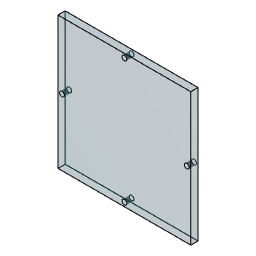
кубсат 2.0 v4 (Autodesk Fusion 360 archive; units mm, degrees)
design "стекло на кубсат 2.0"
Autodesk Fusion 360 part; units mm, degrees
sketch "Sketch1" plane through (0, 0, 0) normal (0, 1, 0) x (1, 0, 0)
  line L0 (-50, -50) -> (33, -50)
  line L1 (33, -50) -> (33, 33)
  line L2 (33, 33) -> (-50, 33)
  line L3 (-50, 33) -> (-50, -50)
  line L4 (-50, -50) -> (-47.5, -50)
  line L5 (-47.5, -50) -> (-47.5, -47.5)
  line L6 (-47.5, -47.5) -> (-50, -47.5)
  line L7 (-50, -47.5) -> (-50, -50)
  line L8 (33, 33) -> (30.5, 33)
  line L9 (30.5, 33) -> (30.5, 30.5)
  line L10 (30.5, 30.5) -> (33, 30.5)
  line L11 (33, 30.5) -> (33, 33)
  line L12 (-47.5, -47.5) -> (30.5, -47.5)
  line L13 (30.5, -47.5) -> (30.5, 30.5)
  line L14 (30.5, 30.5) -> (-47.5, 30.5)
  line L15 (-47.5, 30.5) -> (-47.5, -47.5)
  circle A0 centre (-8.5, -47.5) radius 1.5
  circle A1 centre (-47.5, -8.5) radius 1.5
  circle A2 centre (-8.5, 30.5) radius 1.5
  circle A3 centre (30.5, -8.5) radius 1.5
  dimension "d1" = 83
  dimension "d2" = 83
  dimension "d3" = 2.5
  dimension "d4" = 2.5
  dimension "d5" = 2.5
  dimension "d6" = 2.5
  dimension "d7" = 3
  dimension "d8" = 3
  dimension "d9" = 3
  dimension "d10" = 3
  constraint horizontal L0
  constraint vertical L1
  constraint horizontal L2
  constraint vertical L3
  constraint horizontal L4
  constraint vertical L5
  constraint horizontal L6
  constraint vertical L7
  constraint horizontal L8
  constraint vertical L9
  constraint horizontal L10
  constraint vertical L11
  constraint horizontal L12
  constraint vertical L13
  constraint horizontal L14
  constraint vertical L15
  constraint midpoint L12 A0.centre
  constraint midpoint L15 A1.centre
  constraint midpoint L14 A2.centre
  constraint midpoint L13 A3.centre
  measures "d1" distance of L0.start L0.end
  measures "d2" distance of L0.start L2.end
  measures "d3" distance of L0.start L4.end
  measures "d4" distance of L0.start L6.end
  measures "d5" distance of L1.end L8.end
  measures "d6" distance of L1.end L10.end
  measures "d7" diameter of A0
  measures "d8" diameter of A1
  measures "d9" diameter of A2
  measures "d10" diameter of A3
extrude "Extrude1" add sketch "Sketch1" along normal blind 4.5 contours L0 L3 L4 L5 L6 L7 | L0 L1 L5 L10 L12 L13 A0 A3 | L2 L3 L6 L9 L14 L15 A1 A2 | L12 L13 L14 L15 A0 A1 A2 A3 | L1 L2 L8 L9 L10 L11

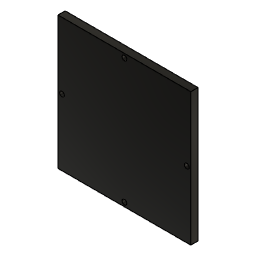
design "стена кубсата"
Autodesk Fusion 360 part; units mm, degrees
sketch "Sketch1" plane through (0, 0, 0) normal (0, 1, 0) x (1, 0, 0)
  line L0 (0, 0) -> (83, 0)
  line L1 (83, 0) -> (83, -83)
  line L2 (83, -83) -> (0, -83)
  line L3 (0, -83) -> (0, 0)
  line L4 (5, -78) -> (78, -78)
  line L5 (78, -78) -> (78, -5)
  line L6 (78, -5) -> (5, -5)
  line L7 (5, -5) -> (5, -78)
  line L8 (5, -78) -> (5, -80.5)
  line L9 (0, -80.5) -> (83, -80.5)
  circle A0 centre (41.5, -80.5) radius 1.5
  line L10 (0, -41.5) -> (26, -41.5)
  line L11 (0, -83) -> (13, -70)
  circle A1 centre (2.5, -41.5) radius 1.5
  line L12 (41.5, -80.5) -> (41.5, -76)
  circle A2 centre (80.5, -41.5) radius 1.5
  circle A3 centre (41.5, -2.5) radius 1.5
  dimension "d1" = 83
  dimension "d2" = 83
  dimension "d3" = 2.5
  dimension "d4" = 3
  constraint horizontal L0
  constraint vertical L1
  constraint horizontal L2
  constraint vertical L3
  constraint coincident L0.start L3.end
  constraint horizontal L4
  constraint vertical L5
  constraint horizontal L6
  constraint vertical L7
  constraint perpendicular L2 L8
  constraint coincident L3 L9.start
  constraint coincident L1 L9.end
  constraint perpendicular L1 L9
  constraint midpoint L9 A0.centre
  constraint midpoint L3 L10.start
  constraint perpendicular L3 L10
  constraint symmetric A0 L11 A1
  constraint coincident A0.centre L12.start
  constraint perpendicular L4 L12
  constraint symmetric A1 L12 A2
  constraint symmetric A0 L10 A3
  measures "d1" distance of L0.start L0.end
  measures "d2" distance of L0.start L2.end
  measures "d3" distance of L4.start L8.end
  measures "d4" diameter of A0
extrude "Extrude1" add sketch "Sketch1" along normal blind 4.5 contours L0 L1 L3 L4 L5 L6 L7 L9 A0 L10 A1 L12 | L3 L7 L9 L10 L11 A1 | L1 L2 L9 A0 L11 | L3 L9 L11 | L8 L9 L11 | L4 L8 L9 A0 L12 | L4 L5 L6 L7

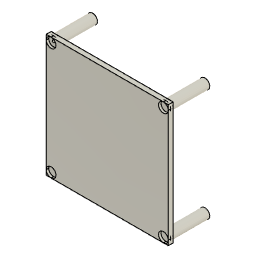
design "Untitled"
Autodesk Fusion 360 part; units mm, degrees
sketch "Sketch1" plane through (0, 0, 0) normal (0, 1, 0) x (1, 0, 0)
  line L0 (-60, -70) -> (-14, -70)
  line L1 (-14, -70) -> (-14, -24)
  line L2 (-14, -24) -> (-60, -24)
  line L3 (-60, -24) -> (-60, -70)
  circle A0 centre (-60, -70) radius 2
  circle A1 centre (-14, -70) radius 2
  circle A2 centre (-60, -24) radius 2
  circle A3 centre (-14, -24) radius 2
  dimension "d1" = 46
  dimension "d2" = 46
  dimension "d3" = 4
  dimension "d4" = 4
  dimension "d5" = 4
  dimension "d6" = 4
  constraint horizontal L0
  constraint vertical L1
  constraint horizontal L2
  constraint vertical L3
  constraint coincident L0.start L3.end
  constraint coincident L0.end L1.start
  constraint coincident L2.end L3.start
  constraint coincident L1.end L2.start
  measures "d1" distance of L0.start L0.end
  measures "d2" distance of L0.start L2.end
  measures "d3" diameter of A0
  measures "d4" diameter of A1
  measures "d5" diameter of A2
  measures "d6" diameter of A3
extrude "Extrude1" add sketch "Sketch1" against normal blind 15 contours L0 L3 A0 | L0 L3 A0 | L0 L1 A1 | L0 L1 A1 | L2 L3 A2 | L2 L3 A2 | L1 L2 A3 | L1 L2 A3 makes body 1 at (-12.1206, -10, 69.316) makes body 2 at (-58.0099, -5, 23.8009) makes body 3 at (-58.0618, -5, 69.5065) makes body 4 at (-12.0099, -10, 24.1991)
sketch "Sketch2" plane through (0, -15, 0) normal (0, -1, 0) x (1, 0, 0)
  circle A0 centre (-60, 70) radius 2
  line L0 (-62, 72) -> (-12, 72)
  line L1 (-12, 72) -> (-12, 22)
  line L2 (-12, 22) -> (-62, 22)
  line L3 (-62, 22) -> (-62, 72)
  constraint horizontal L0
  constraint vertical L1
  constraint horizontal L2
  constraint vertical L3
extrude "Extrude2" add sketch "Sketch2" along normal blind 2 bodies 1 2 3 4
sketch "Sketch3" plane through (0, -17, 0) normal (0, -1, 0) x (1, 0, 0)
  line L0 (-62, 22) -> (-12, 22)
  line L1 (-12, 22) -> (-12, 72)
  line L2 (-12, 72) -> (-62, 72)
  line L3 (-62, 72) -> (-62, 22)
  line L4 (-62, 72) -> (-12, 22)
  line L5 (-62, 72) -> (-59.1716, 69.1716)
  circle A0 centre (-60.5, 70.5) radius 1.5
  circle A1 through (-59.5, 70, -17) (-60.25, 70.433, -17) (-60.25, 69.567, -17)
  dimension "d11" = 4
  dimension "d12" = 1
  constraint coincident L2.end L3.start
  constraint coincident L0.end L1.start
  constraint parallel L4 L5
  constraint coincident L5 A0.centre
  constraint tangent L2 A0
  measures "d11" distance of L2.end L5.end
extrude "Extrude3" cut sketch "Sketch3" along normal blind 59 contours A1 in plane through (0, 0, 0) normal (0, -1, 0) bodies 1
sketch "Sketch4" plane through (0, -17, 0) normal (0, -1, 0) x (1, 0, 0)
  circle A0 centre (-60, 70) radius 0.5
  line L0 (-62, 22) -> (-12, 22)
  line L1 (-12, 22) -> (-12, 72)
  line L2 (-12, 72) -> (-62, 72)
  line L3 (-62, 72) -> (-62, 22)
  circle A1 centre (-60, 70) radius 2
  dimension "d15" = 4
  constraint concentric A0 A1
  measures "d15" diameter of A1
extrude "Extrude4" cut sketch "Sketch4" against normal blind 1 contours A1 bodies 1
sketch "Sketch5" plane through (0, -17, 0) normal (0, -1, 0) x (1, 0, 0)
  arc A0 (-62, 70) -> (-60, 72) centre (-60, 70) ccw
  line L0 (-62, 70) -> (-62, 22)
  line L1 (-62, 22) -> (-12, 22)
  line L2 (-12, 22) -> (-12, 72)
  line L3 (-12, 72) -> (-60, 72)
  circle A1 centre (-60, 70) radius 2
  line L4 (-62, 72) -> (-37, 72)
  line L5 (-37, 72) -> (-37, 61.6718)
  circle A2 centre (-14, 70) radius 2
  line L6 (-62, 72) -> (-62, 47)
  line L7 (-62, 47) -> (-51.7129, 47)
  circle A3 centre (-60, 24) radius 2
  circle A4 centre (-14, 24) radius 2
  dimension "d18" = 25
  dimension "d19" = 25
  constraint concentric A0 A1
  constraint perpendicular L3 L5
  constraint symmetric A1 L5 A2
  constraint perpendicular L0 L7
  constraint symmetric A1 L7 A3
  constraint symmetric A2 L7 A4
  measures "d18" distance of L4.start L4.end
  measures "d19" distance of L4.start L6.end
extrude "Extrude5" cut sketch "Sketch5" against normal blind 1 contours A3 | A2 | A4 bodies 1

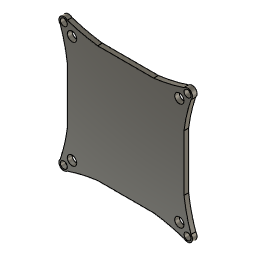
design "основа картриджа под кубсат 2.0"
Autodesk Fusion 360 part; units mm, degrees
sketch "Sketch1" plane through (0, 0, 0) normal (0, 1, 0) x (1, 0, 0)
  line L0 (0, 0) -> (50, 0)
  line L1 (50, 0) -> (50, -50)
  line L2 (50, -50) -> (0, -50)
  line L3 (0, -50) -> (0, 0)
  line L4 (0, -50) -> (-3, -50)
  line L5 (-3, -50) -> (-3, -53)
  line L6 (-3, -53) -> (0, -53)
  line L7 (0, -53) -> (0, -50)
  line L8 (50, 0) -> (53, 0)
  line L9 (53, 0) -> (53, 3)
  line L10 (53, 3) -> (50, 3)
  line L11 (50, 3) -> (50, 0)
  line L12 (0, 0) -> (-3, 0)
  line L13 (-3, 0) -> (-3, 3)
  line L14 (-3, 3) -> (0, 3)
  line L15 (0, 3) -> (0, 0)
  line L16 (50, -50) -> (53, -50)
  line L17 (53, -50) -> (53, -53)
  line L18 (53, -53) -> (50, -53)
  line L19 (50, -53) -> (50, -50)
  arc A0 (13, -50) -> (0, -53) centre (21.5316, -116.6369) ccw
  line L20 (25, -50) -> (25, -32)
  arc A1 (50, -53) -> (37, -50) centre (28.4684, -116.6369) ccw
  line L21 (0, -50) -> (11, -39)
  arc A2 (-3, -50) -> (0, -37) centre (-66.6369, -28.4684) ccw
  arc A3 (50, -37) -> (53, -50) centre (116.6369, -28.4684) ccw
  line L22 (0, -25) -> (30, -25)
  arc A4 (0, -13) -> (-3, 0) centre (-66.6369, -21.5316) ccw
  arc A5 (0, 3) -> (13, 0) centre (21.5316, 66.6369) ccw
  arc A6 (37, 0) -> (50, 3) centre (28.4684, 66.6369) ccw
  line L23 (50, -50) -> (50, 0)
  arc A7 (53, 0) -> (50, -13) centre (116.6369, -21.5316) ccw
  circle A8 centre (-1.5, -51.5) radius 2.1213
  circle A9 centre (-1.5, -51.5) radius 1.5
  circle A10 centre (51.5, -51.5) radius 2.1213
  circle A11 centre (51.5, -51.5) radius 1.5
  circle A12 centre (-1.5, 1.5) radius 1.5
  circle A13 centre (-1.5, 1.5) radius 2.1213
  circle A14 centre (51.5, 1.5) radius 1.5
  circle A15 centre (51.5, 1.5) radius 2.1213
  dimension "d1" = 50
  dimension "d2" = 50
  dimension "d3" = 3
  dimension "d4" = 3
  dimension "d5" = 3
  dimension "d6" = 3
  dimension "d7" = 3
  dimension "d8" = 3
  dimension "d9" = 3
  dimension "d10" = 3
  constraint horizontal L0
  constraint vertical L1
  constraint horizontal L2
  constraint vertical L3
  constraint coincident L0.start L3.end
  constraint horizontal L4
  constraint vertical L5
  constraint horizontal L6
  constraint vertical L7
  constraint horizontal L8
  constraint vertical L9
  constraint horizontal L10
  constraint vertical L11
  constraint horizontal L12
  constraint vertical L13
  constraint horizontal L14
  constraint vertical L15
  constraint horizontal L16
  constraint vertical L17
  constraint horizontal L18
  constraint vertical L19
  constraint coincident L2 A0.start
  constraint midpoint L2 L20.start
  constraint perpendicular L2 L20
  constraint symmetric L6.end L20 L18.end
  constraint symmetric A0.start L20 A1.end
  constraint symmetric A0 L20 A1
  constraint symmetric L6.end L21 L4.end
  constraint symmetric A0.start L21 A2.end
  constraint symmetric A0 L21 A2
  constraint symmetric L20 A2.end A3.start
  constraint symmetric L20 L4.end L16.end
  constraint symmetric L20 A2 A3
  constraint midpoint L3 L22.start
  constraint perpendicular L3 L22
  constraint symmetric L0.end L22 L1.end
  constraint symmetric L1.end L22 L0.end
  constraint symmetric L6.end L22 L14.end
  constraint symmetric A0.start L22 A5.end
  constraint symmetric A0 L22 A5
  constraint symmetric A1.end L22 A6.start
  constraint symmetric L18.end L22 L10.end
  constraint symmetric A1 L22 A6
  constraint symmetric A2.end L22 A4.start
  constraint symmetric L4.end L22 L12.end
  constraint symmetric A2 L22 A4
  constraint symmetric L16.end L22 L8.end
  constraint symmetric A3.start L22 A7.end
  constraint symmetric A3 L22 A7
  constraint coincident L5.end A8
  constraint concentric A8 A9
  constraint tangent L5 A9
  constraint symmetric L20 A8 A10
  constraint symmetric L20 A9 A11
  constraint symmetric L22 A8 A13
  constraint symmetric L22 A9 A12
  constraint symmetric L22 A10 A15
  constraint symmetric L22 A11 A14
  measures "d1" distance of L0.start L0.end
  measures "d2" distance of L0.start L2.end
  measures "d3" distance of L2.end L4.end
  measures "d4" distance of L2.end L6.end
  measures "d5" distance of L0.end L8.end
  measures "d6" distance of L0.end L10.end
  measures "d7" distance of L0.start L12.end
  measures "d8" distance of L0.start L14.end
  measures "d9" distance of L1.end L16.end
  measures "d10" distance of L1.end L18.end
extrude "Extrude1" add sketch "Sketch1" along normal blind 2 contours L0 A5 A13 | L0 L1 L2 L3 L23 | L12 A13 | L12 L15 A12 | L3 A4 A13 | L15 A13 | L12 L13 A12 | L14 L15 A12 | L13 A13 | L0 A6 A15 | L14 A13 | L13 L14 A12 | L1 L23 A7 A15 | L8 L11 A14 | L11 A15 | L8 A15 | L10 A15 | L10 L11 A14 | L3 A2 A8 | L8 L9 A14 | L9 A15 | L9 L10 A14 | L4 L7 A9 | L7 A8 | L2 A0 A8 | L4 A8 | L4 L5 A9 | L5 A8 | L1 A3 L23 A10 | L6 L7 A9 | L5 L6 A9 | L6 A8 | L2 A1 A10 | L16 A10 | L16 L19 A11 | L19 A10 | L16 L17 A11 | L17 A10 | L18 L19 A11 | L18 A10 | L17 L18 A11
sketch "Sketch2" plane through (0, 0, 0) normal (0, 1, 0) x (1, 0, 0)
  circle A0 centre (2, -48) radius 2
  line L0 (25, -50) -> (25, -25)
  line L1 (25, -25) -> (0, -25)
  circle A1 centre (48, -48) radius 2
  circle A2 centre (2, -2) radius 2
  circle A3 centre (48, -2) radius 2
  dimension "d13" = 4
  constraint vertical L0
  constraint perpendicular L0 L1
  constraint symmetric A0 L0 A1
  constraint symmetric A0 L1 A2
  constraint symmetric L1 A1 A3
  measures "d13" diameter of A0
extrude "Extrude2" cut sketch "Sketch2" along normal blind 5
